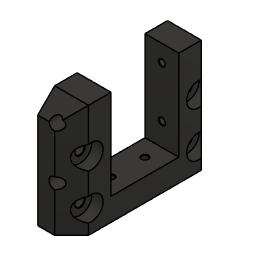
mouse pad stand v1 (Autodesk Fusion 360 archive; units mm, degrees)
design "mousepad stand mount"
Autodesk Fusion 360 part; units mm, degrees
sketch "Sketch1" plane through (0, 0, 0) normal (1, 0, 0) x (0, 0, -1)
  line L0 (-30.1, 40) -> (30.1, 40)
  line L1 (30.1, 40) -> (30.1, -40)
  line L2 (30.1, -40) -> (-30.1, -40)
  line L3 (-30.1, -40) -> (-30.1, 40)
  line L4 (-30.1, 40) -> (30.1, -40) construction
  line L5 (30.1, 40) -> (-30.1, -40) construction
  line L6 (-30.1, 40) -> (-65.1, 40)
  line L7 (-65.1, 40) -> (-65.1, -60)
  line L8 (-65.1, -60) -> (65.1, -60)
  line L9 (65.1, -60) -> (65.1, 40)
  line L10 (65.1, 40) -> (30.1, 40)
  dimension "d1" = 60.2
  dimension "d2" = 80
  dimension "d3" = 35
  dimension "d4" = 20
  constraint horizontal L0
  constraint perpendicular L0 L1
  constraint parallel L0 L2
  constraint parallel L1 L3
  constraint coincident L4 origin
  constraint coincident L5 origin
  constraint perpendicular L3 L6
  constraint perpendicular L6 L7
  constraint perpendicular L7 L8
  constraint perpendicular L6 L9
  constraint perpendicular L1 L10
  constraint equal L6 L10
  measures "d1" distance of L1.end L2.end
  measures "d2" distance of L0.end L1.end
  measures "d3" distance of L0.start L6.end
  measures "d4" distance of L2 L8
extrude "Extrude1" add sketch "Sketch1" along normal blind 30 contours L1 L2 L3 L6 L7 L8 L9 L10 makes body 1
sketch "Sketch2" plane through (0, 0, 0) normal (-1, 0, 0) x (0, 0, 1)
  line L0 (-30.1, 40) -> (-65.1, 40)
  line L1 (-65.1, 40) -> (-65.1, -60)
  line L2 (-65.1, -60) -> (65.1, -60)
  line L3 (65.1, -60) -> (65.1, 40)
  line L4 (65.1, 40) -> (30.1, 40)
  line L5 (30.1, 40) -> (30.1, -40)
  line L6 (30.1, -40) -> (-30.1, -40)
  line L7 (-30.1, -40) -> (-30.1, 40)
  line L8 (-47.6, 40) -> (-47.6, -60) construction
  circle A0 centre (-47.6, -0.3557) radius 10.5
  circle A1 centre (-47.6, -40.3557) radius 10.5
  line L9 (0, 0) -> (0, -40) construction
  circle A2 centre (-47.6, -0.3557) radius 4.25
  circle A3 centre (-47.6, -40.3557) radius 4.25
  circle A4 centre (47.6, -0.3557) radius 10.5
  circle A5 centre (47.6, -0.3557) radius 4.25
  circle A6 centre (47.6, -40.3557) radius 4.25
  circle A7 centre (47.6, -40.3557) radius 10.5
  dimension "d8" = 21
  dimension "d11" = 19.6443
  dimension "d12" = 8.5
  dimension "d13" = 8.5
  dimension "d14" = 40
  constraint midpoint L0 L8.start
  constraint coincident L2 L8.end
  constraint perpendicular L2 L8
  constraint coincident L8 A0.centre
  constraint coincident L8 A1.centre
  constraint equal A0 A1
  constraint coincident L9.start origin
  constraint midpoint L6 L9.end
  constraint concentric A0 A2
  constraint concentric A1 A3
  constraint symmetric A0 L9 A4
  constraint symmetric A1 L9 A7
  constraint symmetric L9 A2 A5
  constraint symmetric L9 A3 A6
  measures "d8" diameter of A0
  measures "d11" distance of L2 A1.centre
  measures "d12" diameter of A2
  measures "d13" diameter of A3
  measures "d14" distance of A0.centre A1.centre
chamfer "Chamfer2" distance 15 angle 45 2 edges at (15, 40, 65.1) (15, 40, -65.1) on bodies 1
chamfer "Chamfer1" distance 15 angle 45 2 edges at (30, -10, 65.1) (30, -10, -65.1) on bodies 1
extrude "Extrude2" cut sketch "Sketch2" against normal blind 60 contours A0 | A1 | A2 | A3 | A4 | A5 | A6 | A7 bodies 1
extrude "Extrude3" add sketch "Sketch2" against normal blind 20 contours A0 | A1 | A4 | A7 bodies 1
sketch "Sketch3" plane through (0, -40, 0) normal (0, 1, 0) x (-1, 0, 0)
  line L0 (0, -30.1) -> (0, 30.1)
  line L1 (0, 30.1) -> (-30, 30.1)
  line L2 (-30, 30.1) -> (-30, -30.1)
  line L3 (-30, -30.1) -> (0, -30.1)
  line L4 (0, 0) -> (-30, 0) construction
  line L5 (-15, 0) -> (-15, 15) construction
  circle A0 centre (-15, 15) radius 5
  circle A1 centre (-15, 15) radius 2.7
  circle A2 centre (-15, -15) radius 5
  circle A3 centre (-15, -15) radius 2.7
  dimension "d20" = 15
  dimension "d21" = 10
  dimension "d22" = 5.4
  constraint coincident L4.start origin
  constraint midpoint L2 L4.end
  constraint midpoint L4 L5.start
  constraint perpendicular L4 L5
  constraint coincident L5.end A0.centre
  constraint concentric A0 A1
  constraint symmetric L4 A0 A2
  constraint symmetric L4 A1 A3
  measures "d20" distance of L5.start L5.end
  measures "d21" diameter of A0
  measures "d22" diameter of A1
extrude "Extrude4" cut sketch "Sketch3" against normal blind 20 contours A0 | A1 | A2 | A3 bodies 1
extrude "Extrude5" add sketch "Sketch3" against normal blind 16 contours A0 | A2 bodies 1
sketch "Sketch4" plane through (0, 0, 30.1) normal (0, 0, -1) x (-1, 0, 0)
  line L0 (0, -40) -> (0, 40)
  line L1 (0, 40) -> (-30, 40)
  line L2 (-30, 40) -> (-30, -40)
  line L3 (-30, -40) -> (0, -40)
  line L4 (-15, 40) -> (-15, -40) construction
  circle A0 centre (-15, 25) radius 5
  circle A1 centre (-15, -20) radius 5
  circle A2 centre (-15, -20) radius 2.7
  circle A3 centre (-15, 25) radius 2.7
  dimension "d27" = 10
  dimension "d28" = 5.4
  dimension "d29" = 15
  dimension "d30" = 20
  constraint midpoint L1 L4.start
  constraint midpoint L3 L4.end
  constraint coincident L4 A0.centre
  constraint coincident L4 A1.centre
  constraint concentric A1 A2
  constraint concentric A0 A3
  constraint equal A0 A1
  constraint equal A2 A3
  measures "d27" diameter of A0
  measures "d28" diameter of A3
  measures "d29" distance of L1 A0.centre
  measures "d30" distance of L3 A1.centre
extrude "Extrude6" cut sketch "Sketch4" along normal blind 150 and the other way blind 65 contours A0 | A1 | A2 | A3 bodies 1
extrude "Extrude7" add sketch "Sketch4" against normal blind 18 contours A0 bodies 1
extrude "Extrude8" add sketch "Sketch4" against normal blind 7 contours A1 bodies 1
extrude "Extrude9" add sketch "Sketch4" along normal blind 18 from surface at 60.2 contours A0 bodies 1
extrude "Extrude10" add sketch "Sketch4" along normal blind 7 from surface at 60.2 contours A1 bodies 1
chamfer "Chamfer3" distance 0.4 angle 45 10 faces at (13.3333, -0.5675, 51.8447) (13.3333, -40.5675, 51.8447) (12.3134, -45.3333, 14.7312) (12.3134, -45.3333, -15.2688) (13.3333, -40.5675, -43.3553) (13.3333, -0.5675, -43.3553) (12.3034, 24.8654, 42.1) (12.3134, -20.2688, 34.7667) (12.3034, 24.8654, -42.1) (12.3134, -20.2688, -34.7667) on bodies 1
copy_body "Body->Comp1" bodies 1 removing the originals makes body 2 in component "mousepad stand mount"
component "mousepad stand mount" placed x (1, 0, 0) y (0, 1, 0) z (0, 0, 1) at (0, 0, 0)
named bodies: "mousepad stand mount"

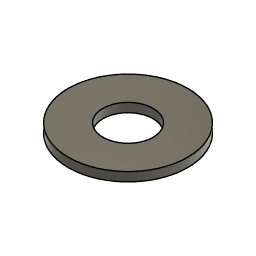
design "M8x20 washer"
Autodesk Fusion 360 part; units mm, degrees
sketch "Sketch1" plane through (0, 0, 0) normal (0, 1, 0) x (1, 0, 0)
  circle A0 centre (0, 0) radius 4.2
  circle A1 centre (0, 0) radius 10
  dimension "d1" = 8.4
  dimension "d2" = 20
  constraint coincident A0.centre A1.centre
  constraint concentric A0 A1
  measures "d1" diameter of A0
  measures "d2" diameter of A1
extrude "Extrude1" add sketch "Sketch1" along normal blind 1.5 makes body 1
copy_body "Body->Comp1" bodies 1 removing the originals makes body 2 in component "M8x20 washer"
component "M8x20 washer" placed x (1, 0, 0) y (0, 1, 0) z (0, 0, 1) at (0, 0, 0)
named bodies: "M8x20 washer"

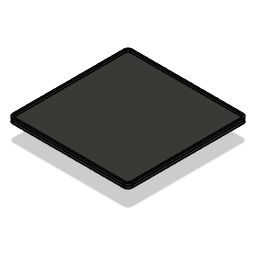
design "mouse pad base"
Autodesk Fusion 360 part; units mm, degrees
sketch "Sketch1" plane through (0, 0, 0) normal (0, 1, 0) x (1, 0, 0)
  line L0 (-110, 110) -> (110, 110)
  line L1 (110, 110) -> (110, -110)
  line L2 (110, -110) -> (-110, -110)
  line L3 (-110, -110) -> (-110, 110)
  line L4 (-110, 110) -> (110, -110) construction
  line L5 (110, 110) -> (-110, -110) construction
  line L6 (107, -107) -> (-107, -107)
  line L7 (-107, -107) -> (-107, 107)
  line L8 (-107, 107) -> (107, 107)
  line L9 (107, 107) -> (107, -107)
  dimension "d1" = 220
  dimension "d2" = 220
  dimension "d3" = 3
  constraint horizontal L0
  constraint perpendicular L0 L1
  constraint parallel L0 L2
  constraint parallel L1 L3
  constraint coincident L4 origin
  constraint coincident L5 origin
  measures "d1" distance of L1.end L2.end
  measures "d2" distance of L0.end L1.end
extrude "Extrude1" add sketch "Sketch1" against normal blind 5 contours L0 L1 L2 L3 | L6 L7 L8 L9 makes body 1
extrude "Extrude2" add sketch "Sketch1" along normal blind 4 separate body makes body 2
sketch "Sketch2" plane through (0, -5, 0) normal (0, -1, 0) x (1, 0, 0)
  line L0 (110, 110) -> (-110, 110)
  line L1 (-110, 110) -> (-110, -110)
  line L2 (-110, -110) -> (110, -110)
  line L3 (110, -110) -> (110, 110)
  line L4 (-50, 30) -> (-50, -30)
  line L5 (-50, 30) -> (60, 30)
  line L6 (60, 30) -> (60, -30)
  line L7 (60, -30) -> (-50, -30)
  dimension "d8" = 60
  dimension "d11" = 30
  dimension "d12" = 60
  dimension "d13" = 110
  constraint vertical L4
  constraint perpendicular L4 L5
  constraint perpendicular L5 L6
  constraint perpendicular L4 L7
  measures "d8" distance of L4.start L4.end
  measures "d11" vertical distance of origin L4.start
  measures "d12" distance of L1 L4
  measures "d13" distance of L4.start L5.end
extrude "Extrude3" add sketch "Sketch2" along normal blind 30 contours L4 L5 L6 L7 bodies 2 1
chamfer "Chamfer1" distance 90 distance2 25 1 edges at (60, -35, 0) measured on face at (-13.3333, -35, 10) on bodies 1
sketch "Sketch3" plane through (-50, 0, 0) normal (-1, 0, 0) x (0, 0, 1)
  line L0 (30, -5) -> (-30, -5)
  line L1 (-30, -5) -> (-30, -35)
  line L2 (-30, -35) -> (30, -35)
  line L3 (30, -35) -> (30, -5)
  line L4 (0, -35) -> (-30, -5) construction
  line L5 (0, -35) -> (30, -5) construction
  circle A0 centre (-15, -20) radius 5
  circle A1 centre (-15, -20) radius 2.7
  circle A2 centre (15, -20) radius 5
  circle A3 centre (15, -20) radius 2.7
  dimension "d18" = 10
  dimension "d19" = 5.4
  constraint midpoint L2 L4.start
  constraint coincident L0.end L1.start
  constraint coincident L0.start L3.end
  constraint midpoint L4 A0.centre
  constraint concentric A0 A1
  constraint midpoint L5 A2.centre
  constraint concentric A2 A3
  constraint equal A1 A3
  constraint equal A0 A2
  measures "d18" diameter of A0
  measures "d19" diameter of A1
extrude "Extrude4" cut sketch "Sketch3" against normal blind 115 contours A0 | A1 | A2 | A3 bodies 1 2
extrude "Extrude5" add sketch "Sketch3" against normal blind 7 contours A0 | A2 bodies 1 2
fillet "Fillet1" radius 7.5 8 edges at (-110, -2.5, 110) (-110, 2, 110) (110, -2.5, 110) (110, 2, 110) (110, -2.5, -110) (110, 2, -110) (-110, -2.5, -110) (-110, 2, -110) on bodies 1 2
fillet "Fillet1" radius 4.5 4 edges at (-107, 2, -107) (-107, 2, 107) (107, 2, 107) (107, 2, -107) on bodies 1 2
chamfer "Chamfer2" distance 1 distance2 1 2 edges at (42, -15, 15) (42, -15, -15) measured on face at (-17.9483, -31.6523, 4.7818) measured on face at (-17.9483, -31.6523, 4.7818) on bodies 1
chamfer "Chamfer2" distance 0.4 distance2 0.4 2 faces at (-45.3333, -20.2688, -12.3134) (-45.3333, -20.2688, 17.6866) on bodies 1
copy_body "Body->Comp1" bodies 1 removing the originals makes body 3 in component "mouse pad base"
copy_body "Body->Comp2" bodies 2 removing the originals makes body 4 in component "mouse pad ridge"
component "mouse pad base" placed x (1, 0, 0) y (0, 1, 0) z (0, 0, 1) at (0, 0, 0)
component "mouse pad ridge" placed x (1, 0, 0) y (0, 1, 0) z (0, 0, 1) at (0, 0, 0)
named bodies: "mouse pad base", "mouse pad ridge"
